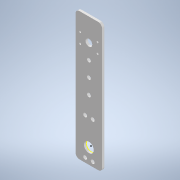
# Autodesk Inventor part: 1
Saved by Autodesk Inventor 2021 (Build 250183000, 183)
## iProperties
Created: 2021-03-30
Part Number: 1
Material: Genérico
Document SubType Name: Modeling
Designer: diego
Density: 1 g/cm^3
Appearance: Valor por defecto
Author: diego
Autodesk Inventor part; units mm, degrees
ref_plane "YZ Plane" through (0, 0, 0) normal (1, 0, 0) x (0, 1, 0)
ref_plane "XZ Plane" through (0, 0, 0) normal (0, 1, 0) x (-1, 0, 0)
ref_plane "XY Plane" through (0, 0, 0) normal (0, 0, 1) x (1, 0, 0)
sketch "Boceto1" plane through (0, 0, 0) normal (0, 0, 1) x (1, 0, 0)
  line L0 (5, 0) -> (30, 0)
  line L1 (35, 5) -> (35, 165)
  line L2 (30, 170) -> (5, 170)
  line L3 (0, 165) -> (0, 5)
  arc A0 (35, 165) -> (30, 170) centre (30, 165) ccw
  arc A1 (5, 170) -> (0, 165) centre (5, 165) ccw
  arc A2 (30, 0) -> (35, 5) centre (30, 5) ccw
  arc A3 (0, 5) -> (5, 0) centre (5, 5) ccw
  constraints: 8 end point, 8 point on circle, 8 tangent, 4 centre point, 3 equal radius, 2 perpendicular, 1 horizontal, 1 vertical
extrude "Extrusión1" add sketch "Boceto1" against normal blind 3
sketch "Boceto2" plane through (0, 0, 0) normal (0, 0, 1) x (1, 0, 0)
  circle A0 centre (17.5, 140) radius 4.5
  circle A1 centre (29, 146.5) radius 1.25
  circle A2 centre (6, 146.5) radius 1.25
  circle A3 centre (6, 133) radius 1.25
  circle A4 centre (29, 133) radius 1.25
  circle A5 centre (17.5, 120) radius 2.5
  circle A6 centre (17.5, 100) radius 2.5
  circle A7 centre (17.5, 80) radius 2.5
  circle A8 centre (17.5, 20) radius 6.5
  circle A9 centre (12.5, 6) radius 2.5
  circle A10 centre (22.5, 6) radius 2.5
  circle A11 centre (12.5, 54.5) radius 2.5
  circle A12 centre (22.5, 54.5) radius 2.5
  point P0 (0, 0)
  constraints: 13 centre point
hole "Agujero1" at (17.5, 140, 0) direction (0, 0, -1) diameter 9 end through all
hole "Agujero2" at (29, 133, 0) at (29, 146.5, 0) at (6, 133, 0) at (6, 146.5, 0) direction (0, 0, -1) diameter 2.5 end through all
hole "Agujero3" at (17.5, 120, 0) at (17.5, 100, 0) at (17.5, 80, 0) at (22.5, 54.5, 0) at (12.5, 54.5, 0) at (22.5, 6, 0) at (12.5, 6, 0) direction (0, 0, -1) diameter 5 end through all
hole "Agujero4" at (17.5, 20, 0) direction (0, 0, -1) diameter 13 end through all
sketch "Boceto3" plane through (0, 0, -3) normal (0, 0, -1) x (-1, 0, 0)
  circle A0 centre (-17.5, 20) radius 6.5 projected
  arc A1 (-27, 23.1225) -> (-8, 23.1225) centre (-17.5, 20) ccw
  line L0 (-17.5, 47) -> (-27, 47)
  line L1 (-17.5, 47) -> (-8, 47)
  line L2 (-8, 47) -> (-8, 23.1225)
  line L3 (-27, 47) -> (-27, 23.1225)
  point P0 (0, 0)
  constraints: 8 end point, 2 point on circle, 1 centre point, 1 coincident, 1 horizontal, 1 parallel, 1 vertical
extrude "Extrusión2" cut sketch "Boceto3" against normal blind 10 contours A0 | L3 L0 L1 L2 A1
